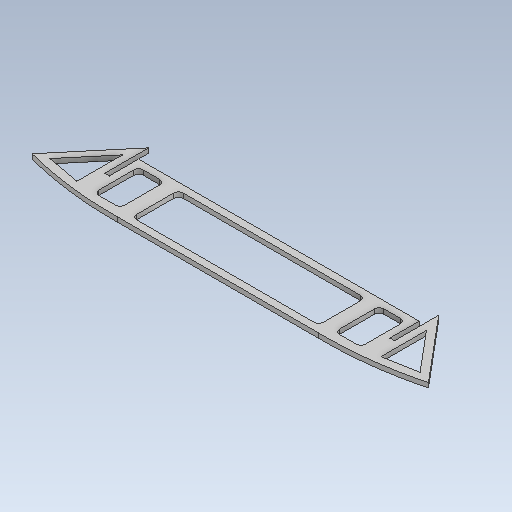
# Autodesk Inventor part: bulkhead_B2
Saved by Autodesk Inventor 2020.3 (Build 243373000, 373)
## iProperties
Created: 2020-05-22
Part Number: bulkhead_B2
Material: Generic
Document SubType Name: Modeling
Designer: kardo
Density: 1 g/cm^3
Appearance: Default
Mass: 3.22284 g
Surface Area: 49.3042 cm^2
Volume: 3.22284 cm^3
Author: kardo
Autodesk Inventor part; units mm, degrees
ref_plane "YZ Plane" through (0, 0, 0) normal (1, 0, 0) x (0, 1, 0)
ref_plane "XZ Plane" through (0, 0, 0) normal (0, 1, 0) x (-1, 0, 0)
ref_plane "XY Plane" through (0, 0, 0) normal (0, 0, 1) x (1, 0, 0)
derived "base_sketch.ipt"
sketch "bulkhead_B2" plane through (0, -204, 0) normal (0, 1, 0) x (-1, 0, 0)
  line L0 (19.176, 46.818) -> (62.322, 46.818)
  line L1 (0, 19.935) -> (28.764, 19.935)
  line L2 (28.764, 13.529) -> (62.322, 13.529)
  line L3 (28.764, 19.935) -> (28.764, 13.529)
  line L4 (62.322, 46.818) -> (62.322, 13.529)
  line L5 (0, 7.65) -> (0, 14.025)
  line L6 (0, 14.025) -> (62.322, 14.025)
  line L7 (0, 7.65) -> (-22.8539, 34.8862)
  line L8 (62.322, 40.0294) -> (19.176, 40.0294)
  line L9 (-19.176, 35.8066) -> (-19.176, 42.5952) construction
  line L10 (-38.352, 36.72) -> (-38.352, 29.9314) construction
  line L11 (19.176, 46.818) -> (19.176, 40.0294) construction
  line L12 (0, 45.9) -> (0, 39.1114) construction
  spline S0 degree 4 poles (-57.528, 27.54) (-46.0483, 34.2051) (-30.6129, 40.5281) (-11.2214, 45.0414) (8.3201, 46.818) (15.5662, 46.818) (19.176, 46.818) knots 0 0 0 0 0 0.630279 0.815816 1 1 1 1 1
  spline S1 degree 3 poles (19.176, 40.0294) (-0.1981, 40.2675) (-19.6083, 37.0145) (-38.352, 29.9314) knots 0 0 0 0 1 1 1 1
  point P0 (0, 0)
ref_plane "bulkhead_B2_plane" through (0, -204, 0) normal (0, 1, 0) x (-1, 0, 0)
sketch "Sketch2" plane through (0, -204, 0) normal (0, 1, 0) x (-1, 0, 0)
  spline S0 degree 3 poles (19.176, 40.0294) (-0.1981, 40.2675) (-19.6083, 37.0145) (-38.352, 29.9314) knots 0 0 0 0 1 1 1 1 projected
  line L0 (62.322, 40.0294) -> (19.176, 40.0294) projected
  line L1 (62.322, 46.818) -> (62.322, 13.529) projected
  line L2 (0, 14.025) -> (62.322, 14.025) projected
  line L3 (0, 7.65) -> (0, 14.025) projected
  line L4 (0, 7.65) -> (-22.8539, 34.8862) projected
  line L5 (-3, 15.8924) -> (-3, 35.5059)
  line L6 (-3, 35.5059) -> (-17.2475, 32.8719)
  line L7 (-17.2475, 32.8719) -> (-3, 15.8924)
  line L8 (7, 36.1114) -> (14.176, 36.1114)
  line L9 (16.176, 34.1114) -> (16.176, 19.025)
  line L10 (14.176, 17.025) -> (7, 17.025)
  line L11 (5, 19.025) -> (5, 34.1114)
  line L12 (24.176, 37.0294) -> (62.322, 37.0294)
  line L13 (62.322, 17.025) -> (24.176, 17.025)
  line L14 (22.176, 19.025) -> (22.176, 35.0294)
  line L15 (0, 14.025) -> (0, 26.5682)
  line L16 (0, 26.5682) -> (2, 26.5682)
  line L17 (2, 26.5682) -> (2, 14.025)
  line L18 (-22.8539, 34.8862) -> (0, 39.1114) construction
  line L19 (0, 39.1114) -> (0, 26.5682) construction
  arc A0 (7, 36.1114) -> (5, 34.1114) centre (7, 34.1114) ccw
  arc A1 (16.176, 34.1114) -> (14.176, 36.1114) centre (14.176, 34.1114) ccw
  arc A2 (14.176, 17.025) -> (16.176, 19.025) centre (14.176, 19.025) ccw
  arc A3 (5, 19.025) -> (7, 17.025) centre (7, 19.025) ccw
  arc A4 (22.176, 19.025) -> (24.176, 17.025) centre (24.176, 19.025) ccw
  arc A5 (24.176, 37.0294) -> (22.176, 35.0294) centre (24.176, 35.0294) ccw
  point P0 (0, 0)
  dimension "d1" = 3
  dimension "d2" = 3
  dimension "d3" = 3
  dimension "d4" = 2
  dimension "d5" = 3
  dimension "d6" = 3
  dimension "d7" = 3
  dimension "d8" = 3
  dimension "d9" = 3
  dimension "d10" = 3
  dimension "d11" = 3
  dimension "d12" = 2
  constraints: 30 end point, 12 point on circle, 12 tangent, 11 parallel, 6 centre point, 5 equal radius, 4 point on line, 2 collinear, 1 perpendicular, 1 vertical, 1 other
  measures "d1" distance between parallel lines of L4 L7
  measures "d2" distance between parallel lines of L18 L6
  measures "d3" distance between parallel lines of L19 L5
  measures "d4" distance between parallel lines of L17 L15
  measures "d5" distance between parallel lines of L17 L11
  measures "d6" distance between parallel lines of L2 L10
  measures "d7" distance from line of L0.end L9
  measures "d8" distance from line of L14 L0.end
  measures "d9" distance between parallel lines of L0 L12
  measures "d10" distance between parallel lines of L2 L13
  measures "d11" distance from line of L18.end L8
  measures "d12" radius of A0
extrude "Extrusion1" add sketch "Sketch2" along normal blind 2 contours L0 L1 L12 A5 L14 A4 L13 L2 L17 L16 L15 L3 L4 S0
mirror "Mirror1" about plane through (-62.322, -204, 14.025) normal (-1, 0, 0) of "Extrusion1"
equation "\"d4\" = stringer_thickness"
equation "\"d13\" = bulkhead_thickness"
equation "\"stringer_thickness\" = 2"
equation "\"bulkhead_thickness\" = 2"
body "Solid1"
